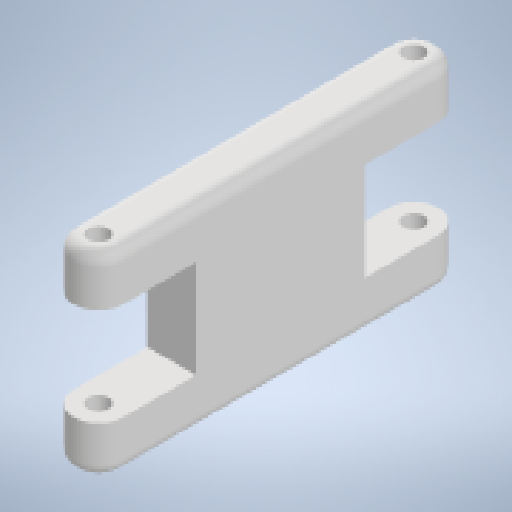
# Autodesk Inventor part: swing pusher
Saved by Autodesk Inventor 2023 (Build 270158000, 158)
## iProperties
Created: 2023-01-25
Part Number: swing pusher
Material: Generic
Document SubType Name: Modeling
Designer: Gabriel - T3 CAD
Density: 1 g/cm^3
Appearance: Default
Mass: 40.324 g
Surface Area: 106.324 cm^2
Volume: 40.324 cm^3
Author: Gabriel - T3 CAD
Autodesk Inventor part; units mm, degrees
ref_plane "YZ Plane" through (0, 0, 0) normal (1, 0, 0) x (0, 1, 0)
ref_plane "XZ Plane" through (0, 0, 0) normal (0, 1, 0) x (-1, 0, 0)
ref_plane "XY Plane" through (0, 0, 0) normal (0, 0, 1) x (1, 0, 0)
sketch "Sketch1" plane through (0, 0, 0) normal (0, 1, 0) x (-1, 0, 0)
  line L0 (0, 0) -> (12.7, 0)
  line L1 (12.7, 0) -> (12.7, 114.3)
  line L2 (12.7, 114.3) -> (0, 114.3)
  line L3 (0, 114.3) -> (0, 0)
  circle A0 centre (6.35, 6.35) radius 2.5797
  circle A1 centre (6.35, 107.95) radius 2.5797
  circle A2 centre (6.35, 6.35) radius 6.35
  circle A3 centre (6.35, 107.95) radius 6.35
  point P0 (0, 107.95)
  point P1 (0, 6.35)
  point P2 (12.7, 6.35)
  point P3 (12.7, 107.95)
  dimension "d0" = 12.7
  dimension "d2" = 6.35
  dimension "d3" = 6.35
  dimension "d4" = 5.1594
  dimension "d5" = 6.35
  dimension "d6" = 5.1594
  dimension "d7" = 6.35
  dimension "d51" = 101.6
  dimension "d52" = 12.7
  dimension "d53" = 12.7
  constraints: 8 end point, 4 centre point, 2 coincident, 2 parallel, 1 horizontal, 1 perpendicular
  measures "d0" distance of L2.end L1.end
  measures "d2" distance from line of L0 A0.centre
  measures "d3" distance from line of L1 A0.centre
  measures "d4" diameter of A0
  measures "d5" distance from line of L1 A1.centre
  measures "d6" diameter of A1
  measures "d7" distance from line of L2 A1.centre
  measures "d51" distance of A0.centre A1.centre
  measures "d52" diameter of A2
  measures "d53" diameter of A3
extrude "Extrusion1" add sketch "Sketch1" along normal blind 50.8 contours A2 | L3 A3 L1 A2 | A3
sketch "Sketch5" plane through (0, 0, 107.95) normal (1, 0, 0) x (0, 0, -1)
  line L0 (107.95, 50.8) -> (101.6, 50.8) projected
  line L1 (0, 0) -> (107.95, 0)
  line L2 (107.95, 0) -> (107.95, 50.8)
  line L3 (107.95, 50.8) -> (0, 50.8)
  line L4 (0, 50.8) -> (0, 0)
  line L5 (107.95, 0) -> (107.95, 50.8) projected
  line L6 (107.95, 38.1) -> (82.55, 38.1)
  line L7 (82.55, 38.1) -> (82.55, 12.7)
  line L8 (82.55, 12.7) -> (107.95, 12.7)
  line L9 (107.95, 12.7) -> (107.95, 38.1)
  line L10 (101.6, 50.8) -> (0, 50.8) projected
  line L11 (-6.35, 0) -> (-6.35, 50.8) projected
  line L12 (0, 50.8) -> (-6.35, 50.8)
  line L13 (-6.35, 50.8) -> (-6.35, 0)
  line L14 (-6.35, 0) -> (0, 0)
  line L15 (0, 0) -> (0, 50.8)
  line L16 (-6.35, 0) -> (-6.35, 50.8) projected
  line L17 (-6.35, 12.7) -> (19.05, 12.7)
  line L18 (19.05, 12.7) -> (19.05, 38.1)
  line L19 (19.05, 38.1) -> (-6.35, 38.1)
  line L20 (-6.35, 38.1) -> (-6.35, 12.7)
  point P0 (95.25, 38.1)
  point P1 (107.95, 38.1)
  dimension "d47" = 25.4
  dimension "d48" = 25.4
  dimension "d49" = 12.7
  constraints: 32 end point, 8 parallel, 4 horizontal, 4 perpendicular, 4 point on line, 2 equal length, 1 collinear, 1 midpoint
  measures "d47" distance of L6.end L7.end
  measures "d48" distance of L6.start L6.end
  measures "d49" distance from line of L10 point (95.25, 38.1)
extrude "Extrusion5" cut sketch "Sketch5" against normal through all contours L2 L8 L7 L6 | L19 L18 L17 L4 | L4 L17 L11 L19
fillet "Fillet3" radius 3.175 24 edges at (-12.7, 38.1, 15.875) (0, 38.1, 15.875) (-6.35, 38.1, 0) (-6.35, 12.7, 0) (-12.7, 12.7, 15.875) (0, 12.7, 15.875) (0, 25.4, 25.4) (-12.7, 25.4, 25.4) (-12.7, 0, 57.15) (-6.35, 0, 114.3) (0, 0, 57.15) (-6.35, 0, 0) (-6.35, 50.8, 114.3) (0, 50.8, 57.15) (-6.35, 50.8, 0) (-12.7, 50.8, 57.15) (0, 25.4, 88.9) (-12.7, 25.4, 88.9) (-6.35, 12.7, 114.3) (-12.7, 12.7, 98.425) (0, 12.7, 98.425) (0, 38.1, 98.425) (-12.7, 38.1, 98.425) (-6.35, 38.1, 114.3)
body "Solid1"
